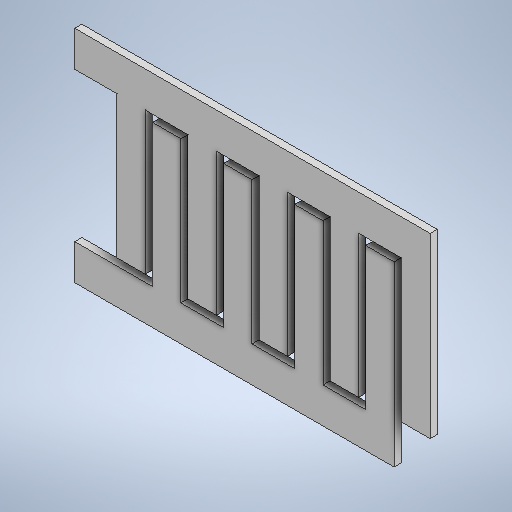
# Autodesk Inventor part: sensor-0001-001
Saved by Autodesk Inventor 2025.2 (Build 292293000, 293)
## iProperties
Created: 2025-01-19
Part Number: sensor-0001-001
Material: Generic
Document SubType Name: Modeling
Designer: kenne
Density: 1 g/cm^3
Appearance: Default
Author: kenne
Autodesk Inventor part; units mm, degrees
ref_plane "YZ Plane" through (0, 0, 0) normal (1, 0, 0) x (0, 1, 0)
ref_plane "XZ Plane" through (0, 0, 0) normal (0, 1, 0) x (-1, 0, 0)
ref_plane "XY Plane" through (0, 0, 0) normal (0, 0, 1) x (1, 0, 0)
sketch "Sketch1" plane through (0, 0, 0) normal (0, 0, 1) x (1, 0, 0)
  line L0 (-21.3826, 17.3138) -> (28.6174, 17.3138)
  line L1 (-21.3826, 17.3138) -> (-21.3826, 12.3138)
  line L2 (28.6174, 17.3138) -> (28.6174, -7.6862)
  line L3 (28.6174, -7.6862) -> (24.6174, -7.6862)
  line L4 (24.6174, -7.6862) -> (24.6174, 12.3138)
  line L5 (24.6174, 12.3138) -> (18.5483, 12.3138)
  line L6 (18.5483, 12.3138) -> (24.5483, 12.3138)
  line L7 (18.5483, 12.3138) -> (18.5483, -7.6862)
  line L8 (18.5483, -7.6862) -> (14.5483, -7.6862)
  line L9 (14.5483, -7.6862) -> (14.5483, 12.3138)
  line L10 (14.5483, 12.3138) -> (8.5483, 12.3138)
  line L11 (8.5483, 12.3138) -> (8.5483, -7.6862)
  line L12 (8.5483, -7.6862) -> (4.5483, -7.6862)
  line L13 (4.5483, -7.6862) -> (4.5483, 12.3138)
  line L14 (4.5483, 12.3138) -> (-1.4517, 12.3138)
  line L15 (-1.4517, 12.3138) -> (-1.4517, -7.6862)
  line L16 (-1.4517, -7.6862) -> (-5.4517, -7.6862)
  line L17 (-5.4517, -7.6862) -> (-5.4517, 12.3138)
  line L18 (-5.4517, 12.3138) -> (-11.4517, 12.3138)
  line L19 (-11.4517, 12.3138) -> (-11.4517, -7.6862)
  line L20 (-11.4517, -7.6862) -> (-15.4517, -7.6862)
  line L21 (-15.4517, -7.6862) -> (-15.4517, 12.3138)
  line L22 (-15.4517, 12.3138) -> (-21.3826, 12.3138)
  line L23 (-21.3826, -13.6862) -> (-21.3826, -8.6862)
  line L24 (-21.3826, -8.6862) -> (-21.3826, -13.6862)
  line L25 (-21.3826, -8.6862) -> (-10.4517, -8.6862)
  line L26 (-10.4517, -8.6862) -> (-10.4517, 11.3138)
  line L27 (-10.4517, 11.3138) -> (-6.4517, 11.3138)
  line L28 (-6.4517, 11.3138) -> (-6.4517, -8.6862)
  line L29 (-6.4517, -8.6862) -> (-0.4517, -8.6862)
  line L30 (-0.4517, -8.6862) -> (-0.4517, 11.3138)
  line L31 (-0.4517, 11.3138) -> (3.5483, 11.3138)
  line L32 (3.5483, 11.3138) -> (3.5483, -8.6862)
  line L33 (3.5483, -8.6862) -> (9.5483, -8.6862)
  line L34 (9.5483, -8.6862) -> (9.5483, 11.3138)
  line L35 (9.5483, 11.3138) -> (13.5483, 11.3138)
  line L36 (13.5483, 11.3138) -> (13.5483, -8.6862)
  line L37 (13.5483, -8.6862) -> (19.5483, -8.6862)
  line L38 (19.5483, -8.6862) -> (19.5483, 11.3138)
  line L39 (19.5483, 11.3138) -> (23.5483, 11.3138)
  line L40 (-21.3826, -13.6862) -> (23.5483, -13.6862)
  line L41 (23.5483, -13.6862) -> (23.5483, 11.3138)
  point P0 (0, 0)
  point P1 (-21.3826, 14.8138)
  point P2 (-21.3826, -11.1862)
  point P3 (-8.4517, 11.3138)
  point P4 (-8.4517, 12.3138)
  point P5 (-18.4171, 12.3138)
  dimension "d1" = 50
  dimension "d2" = 5
  dimension "d3" = 25
  dimension "d4" = 4
  dimension "d5" = 6
  dimension "d6" = 5
  dimension "d22" = 14.8138
  dimension "d23" = 21.3826
  dimension "d24" = 5.9309
  dimension "d25" = 31
  constraints: 84 end point, 21 equal length, 20 perpendicular, 14 point on line, 10 horizontal, 6 vertical, 5 midpoint, 2 vertical alignment, 1 horizontal alignment
  measures "d1" distance of L0.start L0.end
  measures "d2" distance of L0.start L1.end
  measures "d3" distance of L0.end L2.end
  measures "d4" distance of L2.end L3.end
  measures "d5" distance of L5.end L6.end
  measures "d6" distance of L23.end L24.end
  measures "d22" vertical distance of point (0, 0) point (-21.383, 14.814)
  measures "d23" horizontal distance of point (0, 0) point (-21.383, 14.814)
  measures "d24" distance of L21.end L1.end
  measures "d25" distance between parallel lines of L0 L40
extrude "Extrusion1" add sketch "Sketch1" along normal blind 1
body "Solid1"
